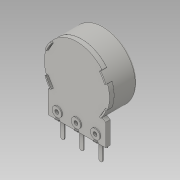
# Autodesk Inventor part: Potenciometro
Saved by Autodesk Inventor 2016 (Build 200138000, 138)
## iProperties
Created: 2018-09-16
Part Number: Potenciometro
Material: Generic
Document SubType Name: Modeling
Designer: Pedro Mendonça
Density: 1 g/cm^3
Appearance: Default
Author: Pedro Mendonça
Autodesk Inventor part; units mm, degrees
ref_plane "YZ Plane" through (0, 0, 0) normal (1, 0, 0) x (0, 1, 0)
ref_plane "XZ Plane" through (0, 0, 0) normal (0, 1, 0) x (-1, 0, 0)
ref_plane "XY Plane" through (0, 0, 0) normal (0, 0, 1) x (1, 0, 0)
sketch "Sketch1" plane through (0, 0, 0) normal (0, 0, 1) x (1, 0, 0)
  line L0 (7.5, -11.75) -> (-7.5, -11.75)
  line L1 (7.5, -11.75) -> (7.5, -5.95)
  line L2 (-7.5, -11.75) -> (-7.5, -5.95)
  line L3 (-7.5, -5.95) -> (-6.2949, -5.2542)
  line L4 (-7.9717, -2.95) -> (-7.7119, -2.8)
  line L5 (-7.4387, -2.8732) -> (-6.2217, -4.981)
  arc A0 (-7.4387, -2.8732) -> (-7.7119, -2.8) centre (-7.6119, -2.9732) ccw
  arc A1 (-6.2949, -5.2542) -> (-6.2217, -4.981) centre (-6.3949, -5.081) ccw
  line L6 (-6.5588, 5.4066) -> (-6.2949, 5.2542)
  line L7 (-7.9717, 2.95) -> (-7.7119, 2.8)
  line L8 (-7.4387, 2.8732) -> (-6.2217, 4.981)
  arc A2 (-7.7119, 2.8) -> (-7.4387, 2.8732) centre (-7.6119, 2.9732) ccw
  arc A3 (-6.2217, 4.981) -> (-6.2949, 5.2542) centre (-6.3949, 5.081) ccw
  line L9 (7.5, -5.95) -> (6.2949, -5.2542)
  line L10 (7.9717, -2.95) -> (7.7119, -2.8)
  line L11 (7.4387, -2.8732) -> (6.2217, -4.981)
  arc A4 (7.7119, -2.8) -> (7.4387, -2.8732) centre (7.6119, -2.9732) ccw
  arc A5 (6.2217, -4.981) -> (6.2949, -5.2542) centre (6.3949, -5.081) ccw
  line L12 (6.5588, 5.4066) -> (6.2949, 5.2542)
  line L13 (7.9717, 2.95) -> (7.7119, 2.8)
  line L14 (7.4387, 2.8732) -> (6.2217, 4.981)
  arc A6 (7.4387, 2.8732) -> (7.7119, 2.8) centre (7.6119, 2.9732) ccw
  arc A7 (6.2949, 5.2542) -> (6.2217, 4.981) centre (6.3949, 5.081) ccw
  arc A8 (-7.9717, 2.95) -> (-7.9717, -2.95) centre (0, 0) ccw
  arc A9 (6.5588, 5.4066) -> (-6.5588, 5.4066) centre (0, 0) ccw
  arc A10 (7.9717, -2.95) -> (7.9717, 2.95) centre (0, 0) ccw
  point P0 (-7.5387, -2.7)
  dimension "d11" = 0.5
  dimension "d12" = 0.2
  dimension "d13" = 0.2
  dimension "d14" = 15
  constraints: 30 end point, 22 point on circle, 11 centre point, 4 tangent, 3 point on line, 1 perpendicular, 1 vertical
  measures "d11" distance of L4.start point (-7.539, -2.7)
  measures "d12" radius of A0
  measures "d13" radius of A1
  measures "d14" distance of L0.start L0.end
extrude "Extrusion1" add sketch "Sketch1" along normal blind 1.2
sketch "Sketch2" plane through (0, 0, 1.2) normal (0, 0, 1) x (1, 0, 0)
  circle A0 centre (-5, -9.75) radius 0.5
  circle A1 centre (0, -9.75) radius 0.5
  circle A2 centre (5, -9.75) radius 0.5
  line L0 (-4.5, -11.55) -> (-4.5, -11.75)
  line L1 (-5.5, -11.55) -> (-5.5, -11.75)
  line L2 (0.5, -11.75) -> (0.5, -11.55)
  line L3 (-0.5, -11.75) -> (-0.5, -11.55)
  line L4 (5.5, -11.55) -> (5.5, -11.75)
  line L5 (4.5, -11.55) -> (4.5, -11.75)
  line L6 (-5.5, -11.75) -> (-5.5, -11.55)
  line L7 (4.5, -11.55) -> (5.5, -11.55)
  line L8 (-5.5, -11.55) -> (-4.5, -11.55)
  line L9 (-0.5, -11.55) -> (0.5, -11.55)
  line L10 (4.5, -11.75) -> (5.5, -11.75)
  line L11 (-5.5, -11.75) -> (-4.5, -11.75)
  line L12 (-0.5, -11.75) -> (0.5, -11.75)
  point P0 (0, 0)
  dimension "d21" = 1
  dimension "d22" = 1
  dimension "d23" = 1
  dimension "d31" = 0.2
  constraints: 26 end point, 3 centre point, 3 horizontal
  measures "d21" diameter of A0
  measures "d22" diameter of A1
  measures "d23" diameter of A2
  measures "d31" distance of L1.start L1.end
extrude "Extrusion2" cut sketch "Sketch2" against normal through all
sketch "Sketch3" plane through (0, 0, 1.2) normal (0, 0, 1) x (1, 0, 0)
  circle A0 centre (-5, -9.75) radius 0.5 projected
  circle A1 centre (-5, -9.75) radius 0.5
  circle A2 centre (-5, -9.75) radius 1.25
  circle A3 centre (0, -9.75) radius 0.5
  circle A4 centre (0, -9.75) radius 1.25
  circle A5 centre (5, -9.75) radius 0.5
  circle A6 centre (5, -9.75) radius 1.25
  circle A7 centre (0, -9.75) radius 0.5
  circle A8 centre (0, -9.75) radius 1.25
  point P0 (0, 0)
  dimension "d34" = 1
  dimension "d35" = 2.5
  dimension "d36" = 1
  dimension "d37" = 2.5
  dimension "d38" = 1
  dimension "d39" = 2.5
  dimension "d40" = 1
  dimension "d41" = 2.5
  constraints: 8 centre point, 5 coincident
  measures "d34" diameter of A1
  measures "d35" diameter of A2
  measures "d36" diameter of A3
  measures "d37" diameter of A4
  measures "d38" diameter of A5
  measures "d39" diameter of A6
  measures "d40" diameter of A7
  measures "d41" diameter of A8
extrude "Extrusion3" add sketch "Sketch3" along normal blind 0.25
sketch "Sketch4" plane through (0, 0, 0) normal (0, 0, -1) x (-1, 0, 0)
  circle A0 centre (-5, -9.75) radius 0.5 projected
  arc A1 (-3.3, -9.75) -> (-6.7, -9.75) centre (-5, -9.75) ccw
  circle A2 centre (-5, -9.75) radius 0.5
  line L0 (-3.3, -9.75) -> (-3.3, -12.75)
  line L1 (-6.7, -9.75) -> (-6.7, -12.75)
  line L2 (-5.5, -11.75) -> (-7.5, -11.75) projected
  line L3 (-6.7, -12.75) -> (-5.5, -12.75)
  line L4 (-4.5, -12.75) -> (-3.3, -12.75)
  arc A3 (-5.5, -16.25) -> (-4.5, -16.25) centre (-5, -16.25) ccw
  line L5 (-4.5, -12.75) -> (-4.5, -16.25)
  line L6 (-5.5, -12.75) -> (-5.5, -16.25)
  line L7 (-5.5, -11.75) -> (-5.5, -11.55) projected
  line L8 (-5.5, -11.55) -> (-4.5, -11.55)
  line L9 (-4.5, -11.55) -> (-4.5, -11.05)
  line L10 (-4.5, -11.05) -> (-5.5, -11.05)
  line L11 (-5.5, -11.05) -> (-5.5, -11.55)
  arc A4 (1.7, -9.75) -> (-1.7, -9.75) centre (0, -9.75) ccw
  circle A5 centre (0, -9.75) radius 0.5
  line L12 (1.7, -9.75) -> (1.7, -12.75)
  line L13 (-1.7, -9.75) -> (-1.7, -12.75)
  line L14 (-1.7, -12.75) -> (-0.5, -12.75)
  line L15 (0.5, -12.75) -> (1.7, -12.75)
  arc A6 (-0.5, -16.25) -> (0.5, -16.25) centre (0, -16.25) ccw
  line L16 (0.5, -12.75) -> (0.5, -16.25)
  line L17 (-0.5, -12.75) -> (-0.5, -16.25)
  line L18 (-0.5, -11.55) -> (0.5, -11.55)
  line L19 (0.5, -11.55) -> (0.5, -11.05)
  line L20 (0.5, -11.05) -> (-0.5, -11.05)
  line L21 (-0.5, -11.05) -> (-0.5, -11.55)
  arc A7 (6.7, -9.75) -> (3.3, -9.75) centre (5, -9.75) ccw
  circle A8 centre (5, -9.75) radius 0.5
  line L22 (6.7, -9.75) -> (6.7, -12.75)
  line L23 (3.3, -9.75) -> (3.3, -12.75)
  line L24 (3.3, -12.75) -> (4.5, -12.75)
  line L25 (5.5, -12.75) -> (6.7, -12.75)
  arc A9 (4.5, -16.25) -> (5.5, -16.25) centre (5, -16.25) ccw
  line L26 (5.5, -12.75) -> (5.5, -16.25)
  line L27 (4.5, -12.75) -> (4.5, -16.25)
  line L28 (4.5, -11.55) -> (5.5, -11.55)
  line L29 (5.5, -11.55) -> (5.5, -11.05)
  line L30 (5.5, -11.05) -> (4.5, -11.05)
  line L31 (4.5, -11.05) -> (4.5, -11.55)
  point P0 (0, 0)
  dimension "d44" = 3.4
  dimension "d45" = 1
  dimension "d52" = 1
  dimension "d53" = 0.5
  dimension "d54" = 3.4
  dimension "d55" = 1
  dimension "d56" = 1
  dimension "d57" = 0.5
  dimension "d58" = 3.4
  dimension "d59" = 1
  dimension "d60" = 1
  dimension "d61" = 0.5
  constraints: 61 end point, 12 point on circle, 9 centre point, 9 perpendicular, 6 parallel, 6 tangent, 3 horizontal, 2 coincident
  measures "d44" diameter of A1
  measures "d45" diameter of A2
  measures "d52" distance of L10.end L9.end
  measures "d53" distance of L9.end L8.end
  measures "d54" diameter of A4
  measures "d55" diameter of A5
  measures "d56" distance of L20.end L19.end
  measures "d57" distance of L19.end L18.end
  measures "d58" diameter of A7
  measures "d59" diameter of A8
  measures "d60" distance of L30.end L29.end
  measures "d61" distance of L29.end L28.end
extrude "Extrusion4" add sketch "Sketch4" along normal blind 0.2
sketch "Sketch5" plane through (0, 0, 0) normal (0, 0, 1) x (1, 0, 0)
  line L0 (-5.5, -11.75) -> (-5.5, -11.55) projected
  line L1 (-5.45, -11.56) -> (-4.55, -11.56)
  line L2 (-4.55, -11.56) -> (-4.55, -11.74)
  line L3 (-4.55, -11.74) -> (-5.45, -11.74)
  line L4 (-5.45, -11.74) -> (-5.45, -11.56)
  line L5 (-0.45, -11.56) -> (0.45, -11.56)
  line L6 (0.45, -11.56) -> (0.45, -11.74)
  line L7 (0.45, -11.74) -> (-0.45, -11.74)
  line L8 (-0.45, -11.74) -> (-0.45, -11.56)
  line L9 (4.55, -11.56) -> (5.45, -11.56)
  line L10 (5.45, -11.56) -> (5.45, -11.74)
  line L11 (5.45, -11.74) -> (4.55, -11.74)
  line L12 (4.55, -11.74) -> (4.55, -11.56)
  point P0 (0, 0)
  dimension "d64" = 0.9
  dimension "d65" = 0.18
  dimension "d70" = 0.9
  dimension "d71" = 0.18
  dimension "d72" = 0.9
  dimension "d73" = 0.18
  constraints: 24 end point, 6 parallel, 3 horizontal, 3 perpendicular
  measures "d64" distance of L2.end L3.end
  measures "d65" distance of L1.end L2.end
  measures "d70" distance of L6.end L7.end
  measures "d71" distance of L5.end L6.end
  measures "d72" distance of L10.end L11.end
  measures "d73" distance of L9.end L10.end
extrude "Extrusion5" add sketch "Sketch5" along normal blind 1.5
sketch "Sketch6" plane through (-0.45, -11.56, 0) normal (0, 1, 0) x (1, 0, 0)
  line L0 (0.9, -1.5) -> (0, -1.5) projected
  line L1 (0.9, -1.5) -> (0, -1.5)
  line L2 (0, -1.5) -> (0, -1.25)
  line L3 (0, -1.25) -> (0.9, -1.25)
  line L4 (0.9, -1.25) -> (0.9, -1.5)
  line L5 (5.9, -1.5) -> (5, -1.5)
  line L6 (5, -1.5) -> (5, -1.25)
  line L7 (5, -1.25) -> (5.9, -1.25)
  line L8 (5.9, -1.25) -> (5.9, -1.5)
  line L9 (-4.1, -1.5) -> (-5, -1.5)
  line L10 (-5, -1.5) -> (-5, -1.25)
  line L11 (-5, -1.25) -> (-4.1, -1.25)
  line L12 (-4.1, -1.25) -> (-4.1, -1.5)
  point P0 (0.45, 0)
  dimension "d76" = 0.25
  dimension "d77" = 0.25
  dimension "d78" = 0.25
  constraints: 24 end point, 6 parallel, 3 horizontal, 3 perpendicular
  measures "d76" distance of L1.end L2.end
  measures "d77" distance of L5.end L6.end
  measures "d78" distance of L9.end L10.end
extrude "Extrusion6" add sketch "Sketch6" along normal blind 0.2
fillet "Fillet1" radius 0.2 6 edges at (-5, -11.74, 1.5) (0, -11.74, 1.5) (5, -11.74, 1.5) (0, -11.74, 0) (-5, -11.74, 0) (5, -11.74, 0)
ref_plane "Work Plane1" through (0, 0, -0.01) normal (0, 0, -1) x (-1, 0, 0)
sketch "Sketch7" plane through (0, 0, -0.01) normal (0, 0, -1) x (-1, 0, 0)
  arc A0 (4.2608, -7.355) -> (-4.2608, -7.355) centre (0, 0) ccw
  line L0 (-4.2608, -7.355) -> (4.2608, -7.355)
  dimension "d83" = 17
  constraints: 2 end point, 2 point on circle, 1 centre point, 1 coincident, 1 horizontal
  measures "d83" diameter of A0
extrude "Extrusion7" add sketch "Sketch7" along normal blind 2
sketch "Sketch8" plane through (0, 0, -2.01) normal (0, 0, -1) x (-1, 0, 0)
  circle A0 centre (0, 0) radius 8.5
  dimension "d86" = 17
  constraints: 1 centre point, 1 coincident
  measures "d86" diameter of A0
extrude "Extrusion8" add sketch "Sketch8" along normal blind 4
fillet "Fillet2" radius 0.5 1 edges at (8.5, 0, -6.01)
sketch "Sketch10" plane through (0, 0, -0.01) normal (0, 0, 1) x (1, 0, 0)
  line L0 (7.9577, -2.9876) -> (7.6063, -2.7847)
  line L1 (7.9577, -2.9876) -> (8.7418, -2.9876) construction
  line L2 (6.605, -5.3501) -> (6.2541, -5.1475)
  line L3 (7.9577, 2.9876) -> (7.6063, 2.7847)
  line L4 (7.9577, 2.9876) -> (8.7418, 2.9876) construction
  line L5 (6.605, 5.3501) -> (6.2541, 5.1475)
  line L6 (-7.9577, -2.9876) -> (-7.6063, -2.7847)
  line L7 (-6.605, -5.3501) -> (-6.2541, -5.1475)
  line L8 (-7.9577, 2.9876) -> (-7.6063, 2.7847)
  line L9 (-6.605, 5.3501) -> (-6.2541, 5.1475)
  arc A0 (7.9577, 2.9876) -> (6.605, 5.3501) centre (0, 0) ccw
  arc A1 (7.6063, 2.7847) -> (6.2541, 5.1475) centre (0, 0) ccw
  arc A2 (-6.2541, 5.1475) -> (-7.6063, 2.7847) centre (0, 0) ccw
  arc A3 (-6.605, 5.3501) -> (-7.9577, 2.9876) centre (0, 0) ccw
  arc A4 (-7.9577, -2.9876) -> (-6.605, -5.3501) centre (0, 0) ccw
  arc A5 (6.5588, -5.4066) -> (7.9577, -2.9876) centre (0, 0) ccw
  arc A6 (-7.6063, -2.7847) -> (-6.2541, -5.1475) centre (0, 0) ccw
  arc A7 (6.2541, -5.1475) -> (7.6063, -2.7847) centre (0, 0) ccw
  point P0 (-6.2949, -5.2542)
  point P1 (-6.2949, 5.2542)
  constraints: 20 end point, 17 point on circle, 8 centre point, 1 coincident, 1 horizontal
extrude "Extrusion9" add sketch "Sketch10" along normal blind 1.6
body "Solid1"
